Autodesk Fusion 360 part; units mm, degrees
note: some values were not read from the file. Chosen so that the rebuilt part matches the saved one: which bodies a step acts on; which face or edge a step refers to. Set by a fixed rule: which sketch regions a step uses.
(part 3 of 3)
sketch "Rear Profile" plane through (0, 0, -104.2517) normal (0, 0, -1) x (-1, 0, 0)
  line L0 (-312.1758, -4) -> (-312.1758, -12)
  line L1 (5.4742, -12) -> (5.4742, -4)
  line L2 (5.4742, -4) -> (-312.1758, -4)
  line L3 (-312.1758, -11.7288) -> (-306.1758, -11.7288)
  line L4 (-306.1758, -11.7288) -> (-306.1758, -23)
  line L5 (-306.1758, -23) -> (-312.1758, -23)
  line L6 (-312.1758, -23) -> (-312.1758, -11.7288)
  line L7 (-0.5258, -11.7288) -> (-0.5258, -23)
  line L8 (5.4742, -23) -> (5.4742, -11.7288)
  line L9 (5.4742, -11.7288) -> (-0.5258, -11.7288)
  line L10 (-0.5258, -23) -> (5.4742, -23)
  line L11 (-312.1758, -12) -> (5.4742, -12)
  line L12 (-312.1758, 7) -> (-312.1758, -4)
  line L13 (-312.1758, -4) -> (5.4742, -4)
  line L14 (5.4742, -4) -> (5.4742, 7)
  line L15 (5.4742, 7) -> (-312.1758, 7)
  line L16 (-0.5258, 0) -> (-306.1758, 0)
  line L17 (-290.8508, -9.5) -> (-286.3508, -9.5)
  line L18 (-281.8508, -9.5) -> (-286.3508, -9.5)
  line L19 (-281.8508, -6) -> (-281.8508, -9.5)
  line L20 (-286.3508, -6) -> (-281.8508, -6)
  line L21 (-286.3508, -6) -> (-290.8508, -6)
  line L22 (-290.8508, -6) -> (-290.8508, -9.5)
  line L23 (-280.8508, -10.5) -> (-286.3508, -10.5)
  line L24 (-291.8508, -10.5) -> (-286.3508, -10.5)
  line L25 (-291.8508, -5) -> (-291.8508, -10.5)
  line L26 (-286.3508, -5) -> (-291.8508, -5)
  line L27 (-286.3508, -5) -> (-280.8508, -5)
  line L28 (-280.8508, -5) -> (-280.8508, -10.5)
  point P0 (5.4742, -19.4575)
extrude "Extrude11" cut sketch "Rear Profile" against normal blind 150 contours L4 L5 L6 L11 | L7 L8 L10 L11 bodies 2
extrude "Extrude13" cut sketch "Rear Profile" against normal blind 20 contours L17 L18 L19 L20 L21 L22 bodies 2
extrude "Extrude12" cut sketch "plate case top view" against normal blind 9.5 contours L0 L491 L492 L499 L544 L545 | L1 L172 L220 L256 L350 L418 L474 L494 | L2 L293 L323 L335 L449 L490 L500 L501 | L3 L21 L26 L115 L207 L216 L413 L424 | L4 L18 L33 L96 L98 L121 L464 L487 | L5 L16 L40 L74 L140 L159 L244 L308 | L6 L52 L53 L67 L117 L147 L154 L164 | L7 L106 L132 L136 L166 L245 L314 L346 | L8 L45 L50 L56 L76 L114 L139 L141 | L9 L34 L58 L69 L135 L152 L189 L438 | L10 L62 L110 L112 L148 L169 L320 L365 | L11 L23 L47 L226 L228 L249 L304 L479 | L12 L82 L84 L88 L100 L124 L156 L163 | L13 L51 L57 L133 L294 L354 L443 L482 | L14 L90 L97 L101 L123 L127 L144 L157 | L15 L19 L27 L44 L49 L89 L102 L125 | L17 L32 L41 L42 L59 L61 L75 L91 | L20 L38 L137 L162 L229 L252 L259 L261 | L22 L54 L93 L95 L150 L364 L478 L486 | L24 L63 L64 L65 L107 L111 L275 L466 | L25 L55 L94 L138 L272 L276 L319 L352 | L28 L43 L113 L168 L269 L306 L383 L404 | L29 L68 L81 L99 L104 L134 L145 L146 | L30 L31 L36 L80 L116 L119 L143 L161 | L35 L39 L71 L86 L126 L130 L131 L142 | L37 L83 L85 L87 L105 L118 L120 L129 | L46 L48 L66 L73 L151 L165 L190 L471 | L60 L185 L186 L224 L351 L399 L434 L436 | L70 L77 L79 L92 L122 L128 L153 L160 | L72 L149 L182 L251 L253 L395 L496 L512 | L78 L103 L155 L158 L210 L222 L290 L296 | L108 L167 L177 L183 L214 L233 L445 L480 | L109 L218 L230 L298 L341 L415 L447 L472 | L170 L215 L311 L339 L348 L427 L437 L469 | L171 L235 L240 L280 L291 L411 L426 L446 | L173 L195 L213 L237 L334 L390 L452 L463 | L174 L202 L239 L242 L312 L374 L378 L435 | L175 L288 L302 L387 L429 L441 L461 L477 | L176 L209 L211 L234 L285 L307 L357 L420 | L178 L180 L258 L268 L277 L366 L386 L484 | L179 L201 L270 L295 L337 L379 L419 L451 | L181 L206 L212 L289 L344 L345 L381 L417 | L184 L194 L198 L303 L313 L407 L456 L485 | L187 L241 L301 L318 L336 L375 L384 L465 | L188 L231 L377 L412 L421 L422 L440 L450 | L191 L385 L388 L400 L403 L405 L430 L460 | L192 L197 L282 L283 L287 L369 L423 L453 | L193 L203 L271 L315 L347 L376 L454 L476 | L196 L221 L266 L292 L382 L398 L428 L467 | L199 L219 L232 L342 L367 L373 L392 L488 | L200 L286 L316 L321 L370 L402 L408 L442 | L204 L297 L300 L358 L360 L389 L439 L481 | L205 L353 L401 L425 L518 L524 | L208 L257 L264 L328 L332 L356 L455 L459 | L217 L236 L248 L262 L267 L338 L368 L394 | L223 L238 L317 L322 L343 L363 L393 L432 | L225 L247 L281 L324 L325 L380 L444 L513 | L227 L250 L273 L305 L406 L431 L498 L509 | L243 L274 L362 L371 L462 L468 L508 L511 | L246 L278 L309 L340 L361 L457 L470 L483 | L254 L263 L326 L327 L329 L510 L562 L563 L564 L573 L581 | L254 L263 L326 L327 L329 L391 L397 L510 L570 L571 L572 L573 L574 L575 L576 L577 L580 L581 | L327 L329 L570 L571 L572 L573 L574 | L327 L329 L562 L573 L574 | L326 L391 L397 L510 L564 L565 L578 L579 L580 L581 | L326 L391 L397 L510 L580 L581 | L327 L329 L562 L574 L576 | L327 L329 L575 L576 L577 | L327 L329 L562 L576 L577 | L327 L329 L391 L397 L562 L565 L577 L580 | L255 L260 L265 L299 L310 L349 L448 L475 | L279 L331 L355 L396 L409 L410 L416 L473 | L284 L330 L333 L458 L489 L497 L506 L514 | L359 L372 L414 L433 L529 L535 | L493 L495 L502 L503 L504 L505 L507 L515 | L516 L517 L519 L520 | L521 L522 L523 L525 | L526 L527 L528 L530 | L531 L532 L533 L534 | L536 L537 L538 L539 | L540 L541 L542 L543 | A0 L547 L549 L551 L553 | A0 L546 L547 L548 L549 | A0 L547 L551 | A0 L549 L553 | A0 L550 L551 L552 L553 | L554 L559 A1 L560 L561 | L554 L555 L558 A1 L560 | L554 L555 A1 | L555 L556 L557 L558 A1 | L558 A1 L560 bodies 2
extrude "Extrude14" cut sketch "Rear Profile" against normal blind 4 contours L23 L24 L25 L26 L27 L28 bodies 2
sketch "Weight and base cuts" plane through (0, -9.5, 0) normal (0, 1, 0) x (-1, 0, 0)
  line L0 (-290.8508, -100.2517) -> (-281.8508, -100.2517)
  line L1 (-281.8508, -100.2517) -> (-281.8508, -98.2517)
  line L2 (-281.8508, -98.2517) -> (-0.5258, -98.2517)
  line L3 (-0.5258, -98.2517) -> (-0.5258, -2.1519)
  line L4 (-0.5258, -2.1519) -> (-306.1758, -2.1519)
  line L5 (-306.1758, -2.1519) -> (-306.1758, -98.2517)
  line L6 (-306.1758, -98.2517) -> (-290.8508, -98.2517)
  line L7 (-290.8508, -98.2517) -> (-290.8508, -100.2517)
  line L8 (-3.3508, -94.2268) -> (-3.3508, -54.2268)
  line L9 (-303.3508, -94.2268) -> (-303.3508, -54.2268)
  line L10 (-3.3508, -94.2268) -> (-303.3508, -94.2268)
  line L11 (-3.3508, -54.2268) -> (-303.3508, -54.2268)
  line L12 (-0.5258, -50.2018) -> (-306.1758, -50.2018)
extrude "Extrude15" cut sketch "Weight and base cuts" against normal blind 4 contours L8 L9 L10 L11 bodies 2
extrude "Extrude16" add sketch "Weight and base cuts" along normal blind 0.5 contours L3 L4 L5 L12 bodies 2
sketch "engrave and split" plane through (0, 7, 0) normal (0, 1, 0) x (-1, 0, 0)
  line L0 (-287.2258, -79.303) -> (-306.1758, -79.303)
  line L1 (-306.1758, -79.303) -> (-306.1758, -2.1519)
  line L2 (-306.1758, -2.1519) -> (-249.1258, -2.1519)
  line L3 (-249.1258, -2.1519) -> (-249.1258, -21.1023)
  line L4 (-249.1258, -21.1023) -> (-239.6008, -21.1023)
  line L5 (-239.6008, -21.1023) -> (-239.6008, -2.1519)
  line L6 (-239.6008, -2.1519) -> (-48.0498, -2.1519)
  line L7 (-48.0498, -2.1519) -> (-48.0498, -21.1023)
  line L8 (-48.0498, -21.1023) -> (-30.0505, -21.1023)
  line L9 (-30.0505, -21.1023) -> (-30.0505, -2.1519)
  line L10 (-30.0505, -2.1519) -> (-0.5258, -2.1519)
  line L11 (-0.5258, -2.1519) -> (-0.5258, -98.2517)
  line L12 (-0.5258, -98.2517) -> (-287.2258, -98.2517)
  line L13 (-287.2258, -98.2517) -> (-287.2258, -79.303)
  line L14 (-312.1758, -104.2517) -> (5.4742, -104.2517)
  line L15 (5.4742, -104.2517) -> (5.4742, 3.8481)
  line L16 (5.4742, 3.8481) -> (-312.1758, 3.8481)
  line L17 (-312.1758, 3.8481) -> (-312.1758, -104.2517)
  line L18 (-306.1758, -79.303) -> (-287.2258, -79.303)
  line L19 (-287.2258, -79.303) -> (-287.2258, -98.2517)
  line L20 (-296.5909, -96.0901) -> (-295.8584, -94.3811)
  spline S0 degree 3 poles (-295.8584, -94.3811) (-295.443, -94.2369) (-294.5672, -93.933) (-294.0438, -93.1642) (-293.7686, -92.76) knots 0 0 0 0 0.128466 0.270828 0.270828 0.270828 0.270828
  spline S1 degree 3 poles (-293.7686, -92.76) (-293.5379, -92.2994) (-293.0771, -91.3794) (-293.0107, -90.3527) (-292.9776, -89.8401) knots 0 0 0 0 0.152852 0.305263 0.305263 0.305263 0.305263
  spline S2 degree 3 poles (-292.9776, -89.8401) (-293.0009, -89.452) (-293.0454, -88.7095) (-293.4688, -88.0998) (-293.6709, -87.8088) knots 0 0 0 0 0.114117 0.218348 0.218348 0.218348 0.218348
  spline S3 degree 3 poles (-293.6709, -87.8088) (-293.9191, -87.5684) (-294.42, -87.0832) (-295.0905, -86.8905) (-295.4288, -86.7932) knots 0 0 0 0 0.101968 0.205808 0.205808 0.205808 0.205808
  line L21 (-295.4288, -86.7932) -> (-296.4541, -91.6174)
  spline S4 degree 3 poles (-296.4541, -91.6174) (-296.5602, -92.111) (-296.7456, -92.9736) (-297.0476, -93.8021) (-297.1768, -94.1565) knots 0 0 0 0 0.151233 0.264264 0.264264 0.264264 0.264264
  spline S5 degree 3 poles (-297.1768, -94.1565) (-297.3107, -94.4298) (-297.5723, -94.9636) (-298.0153, -95.3597) (-298.2315, -95.553) knots 0 0 0 0 0.090331 0.176477 0.176477 0.176477 0.176477
  spline S6 degree 3 poles (-298.2315, -95.553) (-298.4687, -95.7096) (-298.9406, -96.0212) (-299.5041, -96.0672) (-299.7842, -96.0901) knots 0 0 0 0 0.083803 0.166685 0.166685 0.166685 0.166685
  spline S7 degree 3 poles (-299.7842, -96.0901) (-300.1918, -96.037) (-301.0445, -95.9258) (-301.6537, -95.3152) (-301.9717, -94.9963) knots 0 0 0 0 0.11986 0.250793 0.250793 0.250793 0.250793
  spline S8 degree 3 poles (-301.9717, -94.9963) (-302.2504, -94.5756) (-302.8575, -93.6589) (-302.9037, -92.556) (-302.9288, -91.9592) knots 0 0 0 0 0.14861 0.323835 0.323835 0.323835 0.323835
  spline S9 degree 3 poles (-302.9288, -91.9592) (-302.8919, -91.3233) (-302.8191, -90.0686) (-302.2647, -88.9411) (-301.9913, -88.385) knots 0 0 0 0 0.188959 0.372854 0.372854 0.372854 0.372854
  spline S10 degree 3 poles (-301.9913, -88.385) (-301.6879, -87.8983) (-301.1276, -86.9992) (-300.2736, -86.3759) (-299.8819, -86.0901) knots 0 0 0 0 0.170145 0.314283 0.314283 0.314283 0.314283
  spline S11 degree 3 poles (-299.8819, -86.0901) (-299.4425, -85.8849) (-298.4818, -85.4364) (-297.4269, -85.3157) (-296.8545, -85.2502) knots 0 0 0 0 0.144535 0.316001 0.316001 0.316001 0.316001
  line L22 (-296.8545, -85.2502) -> (-296.0831, -81.51)
  line L23 (-296.0831, -81.51) -> (-294.3155, -81.51)
  line L24 (-294.3155, -81.51) -> (-295.087, -85.2502)
  spline S12 degree 3 poles (-295.087, -85.2502) (-294.5088, -85.3792) (-293.3858, -85.6296) (-292.5981, -86.4657) (-292.2159, -86.8713) knots 0 0 0 0 0.173247 0.336542 0.336542 0.336542 0.336542
  spline S13 degree 3 poles (-292.2159, -86.8713) (-291.9225, -87.3453) (-291.3242, -88.3119) (-291.2486, -89.4471) (-291.21, -90.0256) knots 0 0 0 0 0.164552 0.3356 0.3356 0.3356 0.3356
  spline S14 degree 3 poles (-291.21, -90.0256) (-291.2758, -90.7803) (-291.4085, -92.3037) (-292.2891, -93.5546) (-292.7334, -94.1858) knots 0 0 0 0 0.223003 0.450125 0.450125 0.450125 0.450125
  spline S15 degree 3 poles (-292.7334, -94.1858) (-293.2735, -94.7289) (-294.343, -95.8044) (-295.8466, -95.9955) (-296.5909, -96.0901) knots 0 0 0 0 0.222865 0.441322 0.441322 0.441322 0.441322
  spline S16 degree 3 poles (-297.1768, -86.803) (-297.7865, -86.9436) (-298.9962, -87.2228) (-299.7906, -88.1759) (-300.1846, -88.6487) knots 0 0 0 0 0.182287 0.361668 0.361668 0.361668 0.361668
  spline S17 degree 3 poles (-300.1846, -88.6487) (-300.4951, -89.1944) (-301.1208, -90.2943) (-301.2061, -91.5572) (-301.2491, -92.1936) knots 0 0 0 0 0.185755 0.374409 0.374409 0.374409 0.374409
  spline S18 degree 3 poles (-301.2491, -92.1936) (-301.2434, -92.5511) (-301.2334, -93.1833) (-300.9788, -93.7596) (-300.8682, -94.01) knots 0 0 0 0 0.105898 0.187249 0.187249 0.187249 0.187249
  spline S19 degree 3 poles (-300.8682, -94.01) (-300.7401, -94.1922) (-300.4962, -94.5388) (-300.0796, -94.604) (-299.8819, -94.635) knots 0 0 0 0 0.063754 0.121335 0.121335 0.121335 0.121335
  spline S20 degree 3 poles (-299.8819, -94.635) (-299.6842, -94.6068) (-299.2761, -94.5486) (-299.0443, -94.2061) (-298.9248, -94.0295) knots 0 0 0 0 0.057214 0.118079 0.118079 0.118079 0.118079
  spline S21 degree 3 poles (-298.9248, -94.0295) (-298.8044, -93.7372) (-298.4951, -92.987) (-298.3314, -92.1911) (-298.2315, -91.7053) knots 0 0 0 0 0.09467 0.242999 0.242999 0.242999 0.242999
  line L25 (-298.2315, -91.7053) -> (-297.1768, -86.803)
  line L26 (-153.3508, -104.2517) -> (-153.3508, -79)
  line L27 (-153.3508, -79) -> (-163, -79)
  line L28 (-163, -79) -> (-163, -60)
  line L29 (-163, -60) -> (-168, -60)
  line L30 (-168, -60) -> (-168, -41)
  line L31 (-168, -41) -> (-158, -41)
  line L32 (-158, -41) -> (-158, -19)
  line L33 (-158, -19) -> (-190, -19)
  line L34 (-190, -19) -> (-190, 3.8481)
  constraint midpoint L14 L26.start
  constraint perpendicular L12 L26
  constraint perpendicular L26 L27
  constraint perpendicular L12 L28
  constraint perpendicular L28 L29
  constraint perpendicular L29 L30
  constraint perpendicular L30 L31
  constraint perpendicular L6 L32
  constraint perpendicular L32 L33
  constraint coincident L16 L34.end
  constraint perpendicular L16 L34
extrude "Extrude17" cut sketch "engrave and split" against normal blind 0.5 contours L20 S0 S1 S2 S3 L21 S4 S5 S6 S7 S8 S9 S10 S11 L22 L23 L24 S12 S13 S14 S15 bodies 1
split "Split1" by curves path "engrave and split" along L26 L27 L28 L29 L30 L31 L32 L33 L34 bodies 1 2 makes body 4 at (51.4674, -16.0005, -64.7385) makes body 3 at (38.8607, -4, -11.2025)
fillet "Fillet1" radius 2 8 edges at (-5.4742, 1.5, -104.2517) (-5.4742, 1.5, 3.8481) (312.1758, 1.5, -104.2517) (312.1758, 1.5, 3.8481) (-5.4742, -8, -104.2517) (-5.4742, -7, 3.8481) (312.1758, -8, -104.2517) (312.1758, -7, 3.8481) on bodies 1 2 3 4
fillet "Fillet1" radius 1 14 edges at (287.2258, 3.5, -79.303) (306.1758, 3.5, -79.303) (287.2258, 3.5, -98.2517) (306.1758, 3.5, -2.1519) (249.1258, 3.5, -21.1023) (239.6008, 3.5, -21.1023) (239.6008, 3.5, -2.1519) (249.1258, 3.5, -2.1519) (48.0498, 3.5, -2.1519) (48.0498, 3.5, -21.1023) (30.0505, 3.5, -21.1023) (30.0505, 3.5, -2.1519) (0.5258, 3.5, -2.1519) (0.5258, 3.5, -98.2517) on bodies 1 2 3 4
fillet "Fillet1" radius 1.5 4 edges at (290.8508, -6, -99.2517) (281.8508, -6, -99.2517) (281.8508, -9.5, -99.2517) (290.8508, -9.5, -99.2517) on bodies 1 2 3 4
fillet "Fillet1" radius 0.5 4 edges at (280.8508, -5, -102.2517) (280.8508, -10.5, -102.2517) (291.8508, -10.5, -102.2517) (291.8508, -5, -102.2517) on bodies 1 2 3 4
chamfer "Chamfer1" [suppressed]
sketch "bottom pin 1" plane through (153.3508, 0, 0) normal (-1, 0, 0) x (0, 0, 1)
  line L0 (-79, -13.5) -> (-94.2268, -13.5)
  line L1 (-94.2268, -13.5) -> (-94.2268, -9.5)
  line L2 (-94.2268, -9.5) -> (-98.2517, -9.5)
  line L3 (-98.2517, -9.5) -> (-98.2517, -4)
  line L4 (-98.2517, -4) -> (-104.2517, -4)
  line L5 (-104.2517, -4) -> (-104.2517, -12)
  line L6 (-104.2517, -12) -> (-96.2034, -18.7534)
  line L7 (-96.2034, -18.7534) -> (-79, -17.2483)
  line L8 (-79, -17.2483) -> (-79, -13.5)
  circle A0 centre (-98, -13) radius 1.5
  dimension "d117" = 3
  measures "d117" diameter of A0
extrude "Extrude18" cut sketch "bottom pin 1" along normal blind 4 and the other way blind 4 contours A0 bodies 2 4
sketch "bottom pin 2" plane through (168, 0, 0) normal (-1, 0, 0) x (0, 0, 1)
  line L0 (-41, -9) -> (-50.2018, -9)
  line L1 (-50.2018, -9) -> (-50.2018, -9.5)
  line L2 (-50.2018, -9.5) -> (-54.2268, -9.5)
  line L3 (-54.2268, -9.5) -> (-54.2268, -13.5)
  line L4 (-54.2268, -13.5) -> (-60, -13.5)
  line L5 (-60, -13.5) -> (-60, -15.586)
  line L6 (-60, -15.586) -> (-41, -13.9237)
  line L7 (-41, -13.9237) -> (-41, -9)
  circle A0 centre (-48, -12) radius 1
extrude "Extrude20" cut sketch "bottom pin 2" along normal blind 4 and the other way blind 4 contours A0 bodies 2 4
sketch "bottom pin 3" plane through (190, 0, 0) normal (1, 0, 0) x (0, 0, -1)
  line L0 (19, -9) -> (2.1519, -9)
  line L1 (2.1519, -9) -> (2.1519, -4)
  line L2 (2.1519, -4) -> (-3.8481, -4)
  line L3 (-3.8481, -4) -> (-3.8481, -10)
  line L4 (-3.8481, -10) -> (19, -11.9989)
  line L5 (19, -11.9989) -> (19, -9)
  circle A0 centre (-1, -7) radius 1
extrude "Extrude21" cut sketch "bottom pin 3" along normal blind 4 and the other way blind 4000 contours A0 bodies 2 4
sketch "top pin 1" plane through (190, 0, 0) normal (-1, 0, 0) x (0, 0, 1)
  line L0 (-19, -4) -> (3.8481, -4)
  line L1 (3.8481, -4) -> (3.8481, 7)
  line L2 (3.8481, 7) -> (-2.1519, 7)
  line L3 (-2.1519, 7) -> (-2.1519, 0)
  line L4 (-2.1519, 0) -> (-19, 0)
  line L5 (-19, 0) -> (-19, -4)
  circle A0 centre (1, -1) radius 1
extrude "Extrude22" cut sketch "top pin 1" along normal mid plane 8 contours A0 bodies 1 3
sketch "Sketch14" plane through (153.3508, 0, 0) normal (-1, 0, 0) x (0, 0, 1)
  line L0 (-104.2517, -4) -> (-79, -4)
  line L1 (-79, -4) -> (-79, 0)
  line L2 (-79, 0) -> (-98.2517, 0)
  line L3 (-98.2517, 0) -> (-98.2517, 7)
  line L4 (-98.2517, 7) -> (-104.2517, 7)
  line L5 (-104.2517, 7) -> (-104.2517, -4)
  circle A0 centre (-101, -1) radius 1
extrude "Extrude23" cut sketch "Sketch14" along normal mid plane 8 contours A0 bodies 1 3
named bodies: "Top - Right", "Bottom - Right", "Top - Left", "Bottom - Left"
